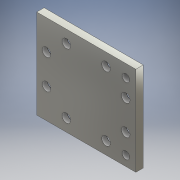
# Autodesk Inventor part: reverse gear steam chest cover
Saved by Autodesk Inventor 2017 (Build 210142000, 142)
## iProperties
Created: 2018-11-06
Part Number: reverse gear steam chest cover
Material: Generic
Document SubType Name: Modeling
Designer: User
Density: 1 g/cm^3
Appearance: Default
Author: User
Autodesk Inventor part; units mm, degrees
ref_plane "YZ Plane" through (0, 0, 0) normal (1, 0, 0) x (0, 1, 0)
ref_plane "XZ Plane" through (0, 0, 0) normal (0, 1, 0) x (-1, 0, 0)
ref_plane "XY Plane" through (0, 0, 0) normal (0, 0, 1) x (1, 0, 0)
sketch "Sketch1" plane through (0, 0, 0) normal (0, 1, 0) x (-1, 0, 0)
  line L0 (0, 0) -> (-40, 0)
  line L1 (-40, 0) -> (-40, -36)
  line L2 (-40, -36) -> (0, -36)
  line L3 (0, -36) -> (0, 0)
  line L4 (0, 0) -> (0, -5)
  circle A0 centre (-12, -5) radius 3
  circle A1 centre (-28, -5) radius 3
  line L5 (0, 0) -> (-4, 0)
  circle A2 centre (-4, -12) radius 3
  line L6 (-40, 0) -> (-36, 0)
  line L7 (-40, -5) -> (-40, 0)
  circle A3 centre (-36, -5) radius 1.5
  circle A4 centre (-4, -24) radius 3
  circle A5 centre (-12, -31) radius 3
  circle A6 centre (-28, -31) radius 3
  circle A7 centre (-36, -32) radius 1.5
  dimension "d0" = 40
  dimension "d1" = 36
  dimension "d11" = 6
  dimension "d13" = 0
  dimension "d14" = 0
  dimension "d15" = 5
  dimension "d16" = 4
  dimension "d17" = 4
  dimension "d18" = 12
  dimension "d19" = 4
  dimension "d20" = 24
  dimension "d21" = 12
  dimension "d22" = 5
  dimension "d23" = 12
  dimension "d24" = 31
  dimension "d25" = 28
  dimension "d26" = 5
  dimension "d27" = 28
  dimension "d29" = 36
  dimension "d30" = 36
  dimension "d31" = 5
  dimension "d32" = 36
  dimension "d34" = 5
  dimension "d88" = 27
  dimension "d89" = 3
  dimension "d90" = 31
  constraints: 16 end point, 8 centre point, 6 equal radius, 3 parallel, 2 horizontal, 2 point on line, 1 perpendicular
  measures "d0" distance of L2.end L1.end
  measures "d1" distance of L1.end L0.end
  measures "d11" diameter of A2
  measures "d13" distance from line of point (0, 0) L4
  measures "d14" distance from line of point (0, 0) L0
  measures "d15" distance from line of L4.end L0
  measures "d16" distance from line of L5.end L4
  measures "d17" distance from line of A2.centre L4
  measures "d18" distance from line of A2.centre L0
  measures "d19" distance from line of A4.centre L4
  measures "d20" distance from line of A4.centre L0
  measures "d21" distance from line of A0.centre L4
  measures "d22" distance from line of A0.centre L0
  measures "d23" distance from line of A5.centre L4
  measures "d24" distance from line of A5.centre L0
  measures "d25" distance from line of A1.centre L4
  measures "d26" distance from line of A1.centre L0
  measures "d27" distance from line of A6.centre L4
  measures "d29" distance from line of L6.end L4
  measures "d30" distance from line of A3.centre L4
  measures "d31" distance from line of A3.centre L0
  measures "d32" distance from line of A7.centre L4
  measures "d34" distance from line of L7.start L0
  measures "d88" distance of A3.centre A7.centre
  measures "d89" diameter of A3
  measures "d90" distance from line of A6.centre L0
extrude "Extrusion1" add sketch "Sketch1" along normal blind 3
sketch "Sketch2" plane through (0, 3, 0) normal (0, 1, 0) x (1, 0, 0)
  line L0 (39.9397, 0) -> (35.9397, 0)
  line L1 (0, 0) -> (40, 0)
  line L2 (35.9397, 0) -> (35.9397, 12)
  line L3 (35.9397, 12) -> (35.9397, 24)
  circle A0 centre (35.9397, 12) radius 3
  circle A1 centre (35.9397, 24) radius 3
  dimension "d4" = 4
  dimension "d5" = 12
  dimension "d6" = 12
  dimension "d7" = 6
  dimension "d8" = 6
  dimension "d35" = 0
  dimension "d36" = 35.9397
  dimension "d37" = 4.0603
  dimension "d38" = 35.9397
  constraints: 8 end point, 2 centre point, 2 coincident, 2 point on line, 1 horizontal, 1 perpendicular, 1 vertical
  measures "d4" distance of L0.start L0.end
  measures "d5" distance of L0.end L2.end
  measures "d6" distance of L2.end L3.end
  measures "d7" diameter of A0
  measures "d8" diameter of A1
  measures "d35" distance from line of point (0, 0) L0
  measures "d36" distance from line of point (0, 0) L2
  measures "d37" distance from line of L1.end L2
  measures "d38" distance from line of L1.start L2
extrude "Extrusion2" cut sketch "Sketch2" against normal blind 3
sketch "Sketch5" plane through (0, 0, 0) normal (0, -1, 0) x (1, 0, 0)
  circle A0 centre (12, -5) radius 1.75
  circle A1 centre (12, -5) radius 3 projected
  circle A2 centre (12, -5) radius 3
  circle A3 centre (28, -5) radius 1.75
  circle A4 centre (28, -5) radius 3 projected
  circle A5 centre (28, -5) radius 3
  circle A6 centre (4, -12) radius 1.75
  circle A7 centre (4, -12) radius 3 projected
  circle A8 centre (4, -12) radius 3
  circle A9 centre (35.9397, -12) radius 1.75
  circle A10 centre (35.9397, -12) radius 3 projected
  circle A11 centre (35.9397, -24) radius 3 projected
  circle A12 centre (28, -31) radius 3 projected
  circle A13 centre (12, -31) radius 3 projected
  circle A14 centre (4, -24) radius 3 projected
  circle A15 centre (4, -12) radius 3 projected
  circle A16 centre (28, -5) radius 3 projected
  circle A17 centre (12, -5) radius 3 projected
  circle A18 centre (36, -32) radius 1.5 projected
  circle A19 centre (36, -5) radius 1.5 projected
  line L0 (0, 0) -> (40, 0) projected
  line L1 (0, -36) -> (0, 0) projected
  line L2 (40, -36) -> (0, -36) projected
  line L3 (40, 0) -> (40, -36) projected
  circle A20 centre (35.9397, -12) radius 3
  circle A21 centre (35.9397, -24) radius 1.75
  circle A22 centre (35.9397, -24) radius 3
  circle A23 centre (28, -31) radius 1.75
  circle A24 centre (28, -31) radius 3
  circle A25 centre (12, -31) radius 1.75
  circle A26 centre (12, -31) radius 3
  circle A27 centre (4, -24) radius 1.75
  circle A28 centre (4, -24) radius 3 projected
  circle A29 centre (4, -24) radius 3
  point P0 (-35.9397, 24)
  point P1 (-28, 31)
  point P2 (-28, 31)
  point P3 (-28, 31)
  dimension "d39" = 3.5
  dimension "d40" = 0
  dimension "d41" = 0
  dimension "d42" = 3.5
  dimension "d43" = 0
  dimension "d44" = 0
  dimension "d45" = 6
  dimension "d46" = 3.5
  dimension "d47" = 0
  dimension "d48" = 0
  dimension "d49" = 6
  dimension "d50" = 3.5
  dimension "d51" = 0
  dimension "d52" = 0
  dimension "d53" = 6
  dimension "d54" = 3.5
  dimension "d55" = 0
  dimension "d56" = 0
  dimension "d57" = 6
  dimension "d58" = 3.5
  dimension "d59" = 0
  dimension "d60" = 0
  dimension "d61" = 6
  dimension "d62" = 3.5
  dimension "d63" = 0
  dimension "d64" = 0
  dimension "d65" = 6
  dimension "d66" = 3.5
  dimension "d67" = 0
  dimension "d68" = 0
  dimension "d69" = 6
  dimension "d74" = 68
  dimension "d75" = 67
  dimension "d76" = 68
  dimension "d77" = 67
  dimension "d78" = 68
  dimension "d79" = 67
  dimension "d80" = 75.9397
  dimension "d81" = 60
  constraints: 16 centre point, 8 coincident, 1 concentric
  measures "d39" diameter of A0
  measures "d40" distance of A1.centre A0.centre
  measures "d41" distance of A1.centre A0.centre
  measures "d42" diameter of A3
  measures "d43" distance of A4.centre A3.centre
  measures "d44" distance of A4.centre A3.centre
  measures "d45" diameter of A5
  measures "d46" diameter of A6
  measures "d47" distance of A7.centre A6.centre
  measures "d48" distance of A7.centre A6.centre
  measures "d49" diameter of A8
  measures "d50" diameter of A9
  measures "d51" distance of A10.centre A9.centre
  measures "d52" distance of A10.centre A9.centre
  measures "d53" diameter of A20
  measures "d54" diameter of A21
  measures "d55" distance of A11.centre A21.centre
  measures "d56" distance of A11.centre A21.centre
  measures "d57" diameter of A22
  measures "d58" diameter of A23
  measures "d59" distance of A12.centre A23.centre
  measures "d60" distance of A12.centre A23.centre
  measures "d61" diameter of A24
  measures "d62" diameter of A25
  measures "d63" distance of A13.centre A25.centre
  measures "d64" distance of A13.centre A25.centre
  measures "d65" diameter of A26
  measures "d66" diameter of A27
  measures "d67" distance of A14.centre A27.centre
  measures "d68" distance of A14.centre A27.centre
  measures "d69" diameter of A29
  measures "d74" distance from line of point (-28, 31) L3
  measures "d75" distance from line of point (-28, 31) L2
  measures "d76" distance from line of point (-28, 31) L3
  measures "d77" distance from line of point (-28, 31) L2
  measures "d78" distance from line of point (-28, 31) L3
  measures "d79" distance from line of point (-28, 31) L2
  measures "d80" distance from line of point (-35.94, 24) L3
  measures "d81" distance from line of point (-35.94, 24) L2
extrude "Extrusion4" add sketch "Sketch5" against normal blind 2 contours A1 | A4 | A7 | A10 | A11 | A12 | A13 | A14
body "Solid1"
